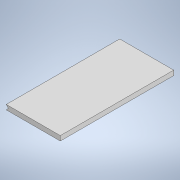
# Autodesk Inventor part: modelGateGate
Saved by Autodesk Inventor 2020 (Build 240168000, 168)
## iProperties
Created: 2023-11-04
Part Number: modelGateGate
Material: Generic
Document SubType Name: Sheet Metal
Designer: jirka
Density: 1 g/cm^3
Sheet Metal Rule: Default_mm
Appearance: Default
Author: jirka
Autodesk Inventor part; units mm, degrees
ref_plane "YZ Plane" through (0, 0, 0) normal (1, 0, 0) x (0, 1, 0)
ref_plane "XZ Plane" through (0, 0, 0) normal (0, 1, 0) x (-1, 0, 0)
ref_plane "XY Plane" through (0, 0, 0) normal (0, 0, 1) x (1, 0, 0)
sketch "Sketch1" plane through (0, 0, 0) normal (0, 1, 0) x (-1, 0, 0)
  line L0 (-20, 42) -> (20, 42)
  line L1 (20, 42) -> (20, -42)
  line L2 (20, -42) -> (-20, -42)
  line L3 (-20, -42) -> (-20, 42)
  point P0 (0, 0)
  dimension "d0" = 40
  dimension "d1" = 84
  dimension "d2" = 20
  dimension "d3" = 42
  constraints: 8 end point, 2 parallel, 1 horizontal, 1 perpendicular
  measures "d0" distance of L1.end L2.end
  measures "d1" distance of L0.end L1.end
  measures "d2" distance from line of point (0, 0) L1
  measures "d3" distance from line of L2 point (0, 0)
extrude "Extrusion1" add sketch "Sketch1" along normal blind 3.5
sketch "Sketch3" plane through (20, 0, -42) normal (0, 0, -1) x (-1, 0, 0)
  line L0 (40, 0) -> (40, 3.5) projected
  line L1 (0, 3.5) -> (40, 3.5) projected
  line L2 (40, 0) -> (38.5, 0)
  line L3 (38.5, 0) -> (38.5, 3.5)
  line L4 (38.5, 3.5) -> (40, 3.5)
  line L5 (40, 3.5) -> (40, 0)
  line L6 (0, 0) -> (40, 0) projected
  line L7 (40, 0) -> (38.5, 1.75)
  line L8 (40, 3.5) -> (38.5, 1.75)
  point P0 (20, 0)
  dimension "d10" = 1.5
  constraints: 12 end point, 2 parallel, 1 horizontal, 1 midpoint, 1 perpendicular, 1 point on line
  measures "d10" distance of L3.end L4.end
extrude "Extrusion2" cut sketch "Sketch3" against normal blind 127.5 contours L7 L8 L0
equation "\"d2\" = 0.5 * d0"
equation "\"d3\" = 0.5 * d1"
equation "\"BendRadius\" = Thickness"
equation "\"BendReliefWidth\" = Thickness"
equation "\"BendReliefDepth\" = 0.5 * Thickness"
equation "\"CornerReliefSize\" = 4 * Thickness"
equation "\"MinimumRemnant\" = 2 * Thickness"
equation "\"TransitionRadius\" = BendRadius"
equation "\"JacobiRadiusSize\" = BendRadius"
equation "\"GapSize\" = Thickness"
equation "\"Thickness\" = 0.5"
body "Solid1"
